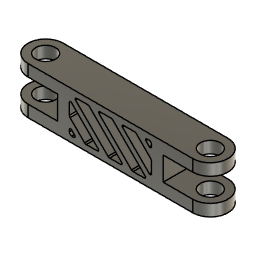
Haste02 v7 (Autodesk Fusion 360 design; units mm, degrees)
Autodesk Fusion 360 part; units mm, degrees
note: some values were not read from the file. Chosen so that the rebuilt part matches the saved one: which bodies a step acts on; which face or edge a step refers to.
sketch "Esboço1" plane through (0, 0, 0) normal (0, 0, 1) x (1, 0, 0)
  circle A0 centre (15, 15) radius 15 construction
  line L0 (1.75, 0) -> (22.5, 0)
  line L1 (0, 1.75) -> (0, 22.5)
  line L2 (15, 30) -> (75, 30)
  line L3 (15, 0) -> (75, 0)
  arc A1 (15, 30) -> (15, 0) centre (15, 15) ccw
  circle A2 centre (15, 15) radius 8.5
  line L4 (75, 30) -> (75, 0)
  circle A3 centre (135, 15) radius 15 construction
  line L5 (135, 0) -> (75, 0)
  line L6 (148.25, 0) -> (127.5, 0)
  circle A4 centre (135, 15) radius 8.5
  line L7 (150, 1.75) -> (150, 22.5)
  arc A5 (135, 0) -> (135, 30) centre (135, 15) ccw
  line L8 (135, 30) -> (75, 30)
  point P0 (150, 0)
  dimension "d1" = 30
  dimension "d2" = 60
  dimension "d3" = 17
  constraint tangent A0 L0
  constraint tangent A0 L1
  constraint coincident A0 L2.start
  constraint tangent A0 L2
  constraint horizontal L2
  constraint coincident A0 L3.start
  constraint parallel L0 L3
  constraint tangent A0 L3
  constraint equal L2 L3
  constraint coincident A0.centre A1.centre
  constraint concentric A1 A2
  constraint symmetric origin L4 P0
  constraint symmetric A0 L4 A3
  constraint symmetric L0.start L4 L6.start
  constraint symmetric L0.end L4 L6.end
  constraint symmetric L1.start L4 L7.start
  constraint symmetric L1.end L4 L7.end
  constraint symmetric L2.start L4 A5.end
  constraint symmetric L2.end L4 L8.end
  constraint symmetric L3.start L4 L5.start
  constraint symmetric L3.end L4 L5.end
  constraint symmetric A1 L4 A5
  constraint symmetric A2 L4 A4
  measures "d1" diameter of A0
  measures "d2" distance of L3.start L3.end
  measures "d3" diameter of A2
extrude "Extrusão1" add sketch "Esboço1" along normal blind 30 makes body 1
extrude "Extrusão2" add 1 faces at (57.8333, 15, 30) along direction (0, 0, 1) blind 10 on bodies 1 bodies 1
sketch "Esboço3" plane through (0, 0, 0) normal (0, -1, 0) x (1, 0, 0)
  line L0 (15, 0) -> (135, 0)
  line L1 (135, 0) -> (135, 40)
  line L2 (135, 40) -> (15, 40)
  line L3 (15, 40) -> (15, 0)
  line L4 (40, 35) -> (110, 35)
  line L5 (110, 35) -> (110, 5)
  line L6 (110, 5) -> (40, 5)
  line L7 (40, 5) -> (40, 35)
  line L8 (40, 35) -> (70, 5) construction
  line L9 (40, 35) -> (82.1616, 35) construction
  line L10 (60, 35) -> (90, 5) construction
  line L11 (80, 35) -> (110, 5) construction
  line L12 (50, 5) -> (40, 15) construction
  line L13 (100, 35) -> (110, 25) construction
  line L14 (40, 31.4645) -> (66.4645, 5)
  line L15 (43.5355, 35) -> (73.5355, 5)
  line L16 (58.5355, 20) -> (55, 16.4645) construction
  line L17 (56.4645, 35) -> (86.4645, 5)
  line L18 (63.5355, 35) -> (93.5355, 5)
  line L19 (76.4645, 35) -> (106.4645, 5)
  line L20 (83.5355, 35) -> (110, 8.5355)
  line L21 (96.4645, 35) -> (110, 21.4645)
  line L22 (103.5355, 35) -> (110, 28.5355)
  line L23 (40, 18.5355) -> (53.5355, 5)
  line L24 (40, 11.4645) -> (46.4645, 5)
  line L25 (40, 20) -> (15, 20)
  line L26 (110, 20) -> (135, 20)
  dimension "d32" = 70
  dimension "d33" = 30
  dimension "d34" = 5
  dimension "d36" = 45
  dimension "d41" = 45
  dimension "d42" = 20
  dimension "d43" = 45
  dimension "d44" = 20
  dimension "d46" = 5
  dimension "d47" = 2.5
  dimension "d48" = 2.5
  dimension "d49" = 2.5
  dimension "d50" = 2.5
  dimension "d51" = 2.5
  dimension "d53" = 2.5
  dimension "d54" = 2.5
  dimension "d55" = 2.5
  dimension "d56" = 2.5
  dimension "d78" = 20
  dimension "d79" = 20
  dimension "d80" = 45
  constraint horizontal L4
  constraint vertical L5
  constraint horizontal L6
  constraint vertical L7
  constraint horizontal L9
  constraint coincident L6 L8.end
  constraint coincident L6 L12.start
  constraint coincident L7 L12.end
  constraint coincident L4 L13.start
  constraint coincident L5 L13.end
  constraint coincident L7 L14.start
  constraint coincident L6 L14.end
  constraint parallel L8 L14
  constraint coincident L4 L15.start
  constraint coincident L6 L15.end
  constraint parallel L8 L15
  constraint midpoint L15 L16.start
  constraint coincident L14 L16.end
  constraint perpendicular L14 L16
  constraint coincident L4 L17.start
  constraint coincident L6 L17.end
  constraint parallel L10 L17
  constraint coincident L4 L18.start
  constraint coincident L6 L18.end
  constraint parallel L10 L18
  constraint coincident L9 L19.start
  constraint parallel L11 L19
  constraint coincident L6 L19.end
  constraint coincident L4 L20.start
  constraint coincident L5 L20.end
  constraint parallel L11 L20
  constraint coincident L4 L21.start
  constraint coincident L4 L22.start
  constraint coincident L5 L22.end
  constraint parallel L13 L22
  constraint parallel L13 L21
  constraint coincident L5 L21.end
  constraint coincident L7 L23.start
  constraint coincident L6 L23.end
  constraint coincident L7 L24.start
  constraint coincident L6 L24.end
  constraint parallel L12 L24
  constraint parallel L12 L23
  constraint coincident L9 L10.start
  constraint coincident L4 L11.start
  constraint coincident L6 L5.end
  constraint coincident L6 L10.end
  constraint coincident L5.end L6.start
  constraint midpoint L7 L25.start
  constraint midpoint L3 L25.end
  constraint midpoint L5 L26.start
  constraint midpoint L1 L26.end
  constraint equal L25 L26
  measures "d32" distance of L4.start L4.end
  measures "d33" distance of L4.start L6.end
  measures "d34" distance of L2 L4
  measures "d36" angle of L8 L9
  measures "d41" angle of L7 L12
  measures "d42" distance of L8.end L12.start
  measures "d43" angle of L4 L13
  measures "d44" distance of L11.start L13.start
  measures "d46" distance of L14 L15
  measures "d47" distance of L8 L15
  measures "d48" distance of L10 L18
  measures "d49" distance of L10 L17
  measures "d50" distance of L11 L20
  measures "d51" distance of L11 L19
  measures "d53" distance of L13 L21
  measures "d54" distance of L13 L22
  measures "d55" distance of L12 L23
  measures "d56" distance of L12 L24
  measures "d78" distance of L4.start L10.start
  measures "d79" distance of L10.start L11.start
  measures "d80" angle of L6 L10
extrude "Extrusão3" cut sketch "Esboço3" against normal through all contours L6 L7 L14 L23 | L4 L5 L20 L21 | L6 L7 L24 | L4 L5 L22 | L4 L6 L15 L17 | L4 L6 L18 L19 bodies 1
fillet "Arredondamento1" radius 1 2 edges at (106.4645, 15, 5) (63.5355, 15, 35) on bodies 1
fillet "Arredondamento2" radius 1 2 edges at (86.4645, 15, 5) (43.5355, 15, 35) on bodies 1
fillet "Arredondamento3" radius 1 2 edges at (40, 15, 31.4645) (66.4645, 15, 5) on bodies 1
fillet "Arredondamento4" radius 1 2 edges at (83.5355, 15, 35) (110, 15, 8.5355) on bodies 1
fillet "Arredondamento5" radius 2 4 edges at (76.4645, 15, 35) (56.4645, 15, 35) (96.4645, 15, 35) (110, 15, 35) on bodies 1
fillet "Arredondamento6" radius 2 4 edges at (93.5355, 15, 5) (73.5355, 15, 5) (53.5355, 15, 5) (40, 15, 5) on bodies 1
fillet "Arredondamento7" radius 2 1 edges at (110, 15, 21.4645) on bodies 1
fillet "Arredondamento8" radius 2 1 edges at (40, 15, 18.5355) on bodies 1
fillet "Arredondamento9" radius 1 2 edges at (40, 15, 11.4645) (46.4645, 15, 5) on bodies 1
fillet "Arredondamento10" radius 1 2 edges at (103.5355, 15, 35) (110, 15, 28.5355) on bodies 1
ref_plane "Plano de trabalho1" through (75, 15, 20) normal (0, 0, 1) x (1, 0, 0)
sketch "Esboço6" plane through (0, 0, 20) normal (0, 0, 1) x (1, 0, 0)
  circle A0 centre (15, 15) radius 15 construction
  line L0 (30, 30.0075) -> (30, 0)
  arc A1 (15, 30) -> (15, 0) centre (15, 15) ccw
  line L1 (15, 30) -> (30, 30.0075)
  line L2 (30, 0) -> (15, 0)
  line L3 (75, 30) -> (75, 0) construction
  arc A2 (135, 0) -> (135, 30) centre (135, 15) ccw
  line L4 (120, 30.0075) -> (120, 0)
  circle A3 centre (135, 15) radius 15 construction
  line L5 (135, 30) -> (120, 30.0075)
  line L6 (120, 0) -> (135, 0)
  point P0 (150, 0)
  constraint vertical L0
  constraint tangent A0 L0
  constraint coincident A0 A1.end
  constraint coincident A0 A1.start
  constraint coincident A0.centre A1.centre
  constraint tangent A1 L2
  constraint parallel L0 L3
  constraint symmetric origin L3 P0
  constraint symmetric A0 L3 A3
  constraint symmetric L0.start L3 L4.start
  constraint symmetric L0.end L3 L4.end
  constraint symmetric A1.start L3 A2.end
  constraint symmetric A1.end L3 A2.start
  constraint symmetric A1 L3 A2
extrude "Extrusão4" cut sketch "Esboço6" along normal mid plane 20 bodies 1
scale "Escala1" factor 0.588235 about (135, 30, 40) bodies 1
ref_plane "Plano de trabalho2" through (126.1765, 21.1765, 28.2353) normal (1, 0, 0) x (0, 1, 0)
split "Dividir1" by plane through (126.1765, 21.1765, 28.2353) normal (1, 0, 0) bodies 1 makes body 2 at (127.451, 21.1765, 34.1176) makes body 3 at (127.451, 21.1765, 22.3529)
move_body "Mover1" bodies 3 2 to x (1, 0, 0) y (0, 1, 0) z (0, 0, 1) at (6, 0, 0)
extrude "Extrusão5" add 2 faces at (132.1765, 18.2353, 36.0784) (132.1765, 18.2353, 18.4314) along direction (-1, 0, 0) up to surface end surface through (126.1765, 30.0044, 28.2353) normal (1, 0, 0) offset 0 on bodies 2 3 bodies 1 2 3
ref_plane "Plano de trabalho3" through (73.2353, 21.1765, 28.2353) normal (-1, 0, 0) x (0, -1, 0)
split "Dividir2" by plane through (73.2353, 21.1765, 28.2353) normal (-1, 0, 0) bodies 1 makes body 4 at (71.9608, 21.1765, 40) makes body 5 at (71.9608, 21.1765, 16.4706)
move_body "Mover2" bodies 4 5 to x (1, 0, 0) y (0, 1, 0) z (0, 0, 1) at (-6, 0, 0)
extrude "Extrusão6" add 2 faces at (67.2353, 18.2353, 38.0392) (67.2353, 18.2353, 20.3922) along direction (1, 0, 0) up to near side of body 1 on bodies 4 5 bodies 1 4 5
equation "d84 = 10 / 17"
